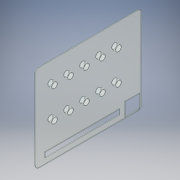
# Autodesk Inventor part: frount glass
Saved by Autodesk Inventor 2019 (Build 230136000, 136)
## iProperties
Created: 2020-03-10
Part Number: frount glass
Material: Glass
Document SubType Name: Modeling
Designer: Hp
Density: 2.18 g/cm^3
Appearance: Clear
Author: Hp
Autodesk Inventor part; units mm, degrees
ref_plane "YZ Plane" through (0, 0, 0) normal (1, 0, 0) x (0, 1, 0)
ref_plane "XZ Plane" through (0, 0, 0) normal (0, 1, 0) x (-1, 0, 0)
ref_plane "XY Plane" through (0, 0, 0) normal (0, 0, 1) x (1, 0, 0)
sketch "Sketch1" plane through (0, 0, 0) normal (1, 0, 0) x (0, 1, 0)
  line L0 (0, 0) -> (245, 0)
  line L1 (245, 0) -> (245, -298.222)
  line L2 (245, -298.222) -> (0, -298.222)
  line L3 (0, -298.222) -> (0, 0)
  dimension "d0" = 245
  dimension "d1" = 298.222
  constraints: 8 end point, 2 parallel, 1 horizontal, 1 perpendicular
  measures "d0" distance of L1.end L2.end
  measures "d1" distance of L0.end L1.end
extrude "Extrusion1" add sketch "Sketch1" along normal blind 2
sketch "Sketch2" plane through (2, 0, 0) normal (1, 0, 0) x (0, 0, -1)
  line L0 (252.355, 2) -> (293.422, 2)
  line L1 (293.422, 2) -> (293.422, 40)
  line L2 (293.422, 40) -> (252.355, 40)
  line L3 (252.355, 40) -> (252.355, 2)
  line L4 (0, 0) -> (298.222, 0) projected
  line L5 (0, 245) -> (0, 0) projected
  line L6 (298.222, 0) -> (298.222, 245) projected
  dimension "d4" = 2
  dimension "d6" = 38
  dimension "d7" = 41.067
  dimension "d8" = 4.8
  constraints: 8 end point, 2 parallel, 1 horizontal, 1 perpendicular
  measures "d4" distance between parallel lines of L0 L4
  measures "d6" distance of L0.end L1.end
  measures "d7" distance of L0.start L0.end
  measures "d8" distance between parallel lines of L6 L1
extrude "Extrusion2" cut sketch "Sketch2" against normal blind 10
sketch "Sketch3" plane through (2, 0, 0) normal (1, 0, 0) x (0, 0, -1)
  line L0 (237.355, 29.8) -> (27, 29.8)
  line L1 (27, 29.8) -> (27, 15.8)
  line L2 (27, 15.8) -> (237.355, 15.8)
  line L3 (237.355, 15.8) -> (237.355, 29.8)
  line L4 (252.355, 2) -> (252.355, 40) projected
  line L5 (0, 0) -> (298.222, 0) projected
  line L6 (0, 245) -> (0, 0) projected
  dimension "d11" = 15
  dimension "d12" = 15.8
  dimension "d13" = 14
  dimension "d14" = 27
  constraints: 8 end point, 2 parallel, 1 horizontal, 1 perpendicular
  measures "d11" distance between parallel lines of L4 L3
  measures "d12" distance between parallel lines of L5 L2
  measures "d13" distance of L2.end L0.start
  measures "d14" distance between parallel lines of L6 L1
extrude "Extrusion3" cut sketch "Sketch3" against normal blind 10
sketch "Sketch4" plane through (0, 0, 0) normal (-1, 0, 0) x (0, 0, 1)
  circle A0 centre (-223.222, 190) radius 7.5
  line L0 (0, 245) -> (-298.222, 245) projected
  line L1 (-298.222, 245) -> (-298.222, 0) projected
  point P0 (0, 0)
  dimension "d17" = 15
  dimension "d18" = 55
  dimension "d19" = 75
  constraints: 1 centre point
  measures "d17" diameter of A0
  measures "d18" distance from line of L0 A0.centre
  measures "d19" distance from line of L1 A0.centre
extrude "Extrusion4" cut sketch "Sketch4" against normal blind 10
pattern_linear "Rectangular Pattern1" count 5 spacing 45 along (0, 0, 1) of "Extrusion4"
pattern_linear "Rectangular Pattern2" count 2 spacing 86.16 along (0, -1, 0) of "Extrusion4", "Rectangular Pattern1"
sketch "Sketch5" plane through (2, 0, 0) normal (1, 0, 0) x (0, 0, -1)
  circle A0 centre (43.222, 190) radius 7.5 projected
  circle A1 centre (43.222, 190) radius 7.5
  circle A2 centre (43.222, 190) radius 8.5
  point P0 (0, 0)
  dimension "d28" = 17
  constraints: 2 centre point, 2 coincident
  measures "d28" diameter of A2
extrude "Extrusion5" add sketch "Sketch5" along normal blind 10
pattern_linear "Rectangular Pattern3" count 5 spacing 45 along (0, 0, -1) of "Extrusion5"
pattern_linear "Rectangular Pattern4" count 2 spacing 86.16 along (0, -1, 0) of "Extrusion5", "Rectangular Pattern3"
fillet "Fillet1" radius 10 4 edges at (1, 245, 0) (1, 245, -298.222) (1, 0, -298.222) (1, 0, 0)
body "Solid1"
